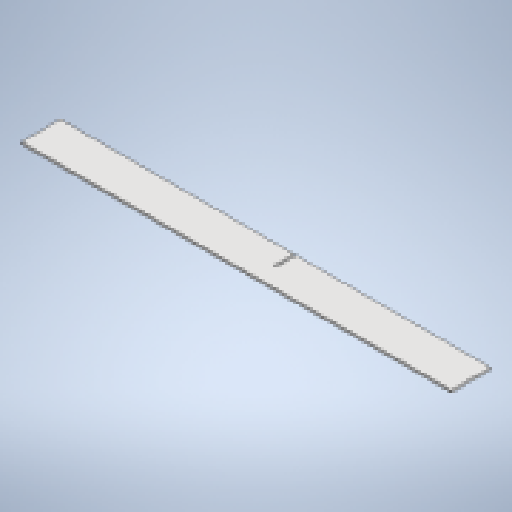
# Autodesk Inventor part: BSH 042 stringer floor
Saved by Autodesk Inventor 2025 (Build 290162010, 162A)
## iProperties
Created: 2024-07-23
Part Number: BSH 042 stringer floor
Material: 09g2s
Document SubType Name: Sheet Metal
Designer: pokla
Mass: 5330.4 g
Surface Area: 4696.25 cm^2
Volume: 679.031 cm^3
Density: 7.85 g/cm^3
Flat Pattern Width: 5 cm
Flat Pattern Length: 55.02 cm
Flat Pattern Area: 275.1 cm^2
Sheet Metal Rule: AISI304 3mm Die 32
Sheet Metal Width: 50,000 mm
Sheet Metal Length: 550,200 mm
Sheet Metal Area: 27510,000 mm^2
Appearance: Default
Author: admin
Autodesk Inventor part; units mm, degrees
ref_plane "YZ Plane" through (0, 0, 0) normal (1, 0, 0) x (0, 1, 0)
ref_plane "XZ Plane" through (0, 0, 0) normal (0, 1, 0) x (-1, 0, 0)
ref_plane "XY Plane" through (0, 0, 0) normal (0, 0, 1) x (1, 0, 0)
sketch "Sketch8" plane through (0, 0, 0) normal (0, 0, 1) x (1, 0, 0)
  line L0 (-275.1, 50) -> (275.1, 50)
  line L1 (275.1, 50) -> (275.1, 0)
  line L2 (275.1, 0) -> (-275.1, 0)
  line L3 (-275.1, 0) -> (-275.1, 50)
  point P0 (0, 0)
  point P1 (0, 0)
  dimension "d37" = 50
  dimension "d38" = 550.2
  measures "d37" distance of L0.end L1.end
  measures "d38" distance of L0.start L0.end
extrude "Plate5" add sketch "Sketch8" against normal blind 3
sketch "Sketch9" plane through (0, 0, 0) normal (0, 0, 1) x (1, 0, 0)
  line L0 (275.1, 50) -> (-275.1, 50) projected
  line L1 (23.5, 50) -> (26.7, 50)
  line L2 (26.7, 50) -> (26.7, 24)
  line L3 (26.7, 24) -> (23.5, 24)
  line L4 (23.5, 24) -> (23.5, 50)
  line L5 (-275.1, 50) -> (-275.1, 0) projected
  point P0 (0, 0)
  point P1 (26.7, 50)
  dimension "d42" = 298.6
  dimension "d43" = 3.2
  dimension "d44" = 26
  constraints: 8 end point, 2 parallel, 1 horizontal, 1 perpendicular, 1 point on line
  measures "d42" distance between parallel lines of L4 L5
  measures "d43" distance between parallel lines of L4 L2
  measures "d44" distance of L1.end L2.end
extrude "Extrusion3" cut sketch "Sketch9" against normal through all
equation "\"d41\" = Thickness"
equation "\"BendReliefWidth\" = Thickness"
equation "\"BendReliefDepth\" = 0.5 * Thickness"
equation "\"CornerReliefSize\" = 4 * Thickness"
equation "\"MinimumRemnant\" = 2 * Thickness"
equation "\"TransitionRadius\" = BendRadius"
equation "\"JacobiRadiusSize\" = BendRadius"
equation "\"GapSize\" = Thickness"
equation "\"Thickness\" = 3"
equation "\"BendRadius\" = 5"
body "Solid3"
